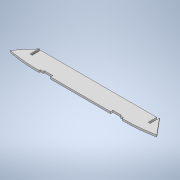
# Autodesk Inventor part: transom
Saved by Autodesk Inventor 2020.3 (Build 243373010, 373A)
## iProperties
Created: 2020-05-22
Part Number: transom
Material: Generic
Document SubType Name: Modeling
Designer: kardo
Density: 1 g/cm^3
Appearance: Default
Mass: 5.00225 g
Surface Area: 57.3573 cm^2
Volume: 5.00225 cm^3
Author: kardo
Autodesk Inventor part; units mm, degrees
ref_plane "YZ Plane" through (0, 0, 0) normal (1, 0, 0) x (0, 1, 0)
ref_plane "XZ Plane" through (0, 0, 0) normal (0, 1, 0) x (-1, 0, 0)
ref_plane "XY Plane" through (0, 0, 0) normal (0, 0, 1) x (1, 0, 0)
derived "base_sketch.ipt"
sketch "transom" plane through (0, -306, 31.875) normal (0, 1, 0) x (-1, 0, 0)
  line L0 (19.176, 14.943) -> (62.322, 14.943)
  line L1 (62.322, 14.943) -> (62.322, -18.346)
  line L2 (28.764, -18.346) -> (62.322, -18.346)
  line L3 (0, -18.5331) -> (-13.7575, -2.1376)
  line L4 (0, -18.5331) -> (0, -17.85)
  line L5 (0, -17.85) -> (62.322, -17.85)
  line L6 (62.322, 0.918) -> (19.176, 0.918)
  line L7 (19.176, 14.943) -> (19.176, 0.918) construction
  line L8 (-2.8595, -0.3503) -> (-2.8595, 13.6747) construction
  line L9 (-13.7575, 11.8874) -> (-13.7575, -2.1376) construction
  line L10 (8.1347, 14.7187) -> (8.1347, 0.6937) construction
  spline S0 degree 4 poles (-57.528, -4.335) (-46.0483, 2.3301) (-30.6129, 8.6531) (-11.2214, 13.1664) (8.3201, 14.943) (15.5662, 14.943) (19.176, 14.943) knots 0 0 0 0 0 0.630279 0.815816 1 1 1 1 1
  spline S1 degree 3 poles (19.176, 0.918) (8.1274, 1.1291) (-2.9238, -0.0043) (-13.7575, -2.1376) knots 0 0 0 0 1 1 1 1
  line L11 (0, 0) -> (0, -20.4)
  line L12 (0, 0) -> (0, 14.025) construction
  line L13 (-13.7575, 11.8874) -> (-2.8595, 13.6747) construction
  line L14 (-2.8595, 13.6747) -> (8.1347, 14.7187) construction
  line L15 (8.1347, 14.7187) -> (19.176, 14.943) construction
  point P0 (0, -31.875)
  point P1 (-38.352, -9.18)
  point P2 (-19.176, 10.7202)
  point P3 (-38.352, 4.845)
ref_plane "transom_plane" through (0, -306, 31.875) normal (0, 1, 0) x (-1, 0, 0)
sketch "Sketch2" plane through (0, -306, 31.875) normal (0, 1, 0) x (-1, 0, 0)
  line L0 (0, -18.5331) -> (-13.7575, -2.1376) projected
  line L1 (0, -17.85) -> (62.322, -17.85) projected
  line L2 (0, -20.4) -> (0, -17.85) projected
  spline S0 degree 3 poles (19.176, 0.918) (8.1274, 1.1291) (-2.9238, -0.0043) (-13.7575, -2.1376) knots 0 0 0 0 1 1 1 1 projected
  line L3 (62.322, 0.918) -> (19.176, 0.918) projected
  line L4 (62.322, 14.943) -> (62.322, -18.346) projected
  line L5 (0, -17.85) -> (0, -8.9267)
  line L6 (0, -8.9267) -> (2, -8.9267)
  line L7 (2, -8.9267) -> (2, -17.85)
  line L8 (0, -8.9267) -> (0, -0.0034) construction
  line L9 (19.176, 0.918) -> (19.176, -0.282)
  line L10 (19.176, -0.282) -> (22.176, -0.282)
  line L11 (22.176, -0.282) -> (25.176, -0.282) construction
  line L12 (25.176, -0.282) -> (25.176, 0.918) construction
  line L13 (22.176, -0.282) -> (22.176, -1.482)
  line L14 (22.176, -1.482) -> (31.176, -1.482)
  line L15 (31.176, -1.482) -> (31.176, 0.918)
  point P0 (0, -31.875)
  point P1 (-38.352, -9.18)
  dimension "d1" = 2
  dimension "d4" = 1.2
  dimension "d5" = 1.2
  dimension "d6" = 6
  dimension "d7" = 6
  constraints: 22 end point, 5 parallel, 4 collinear, 4 perpendicular, 3 point on line, 2 other
  measures "d1" distance of L5.end L6.end
  measures "d4" distance of L3.end L9.end
  measures "d5" distance of L10.end L13.end
  measures "d6" distance between parallel lines of L9 L12
  measures "d7" distance between parallel lines of L15 L12
extrude "Extrusion1" add sketch "Sketch2" along normal blind 2 contours L0 S0 L9 L10 L13 L14 L15 L3 L4 L1 L7 L6 L5 L2
mirror "Mirror1" about plane through (-62.322, -306, 14.025) normal (-1, 0, 0) of "Extrusion1"
equation "\"d1\" = stringer_thickness"
equation "\"d4\" = decking_thickness"
equation "\"d5\" = decking_thickness"
equation "\"d6\" = cowl_strip_width"
equation "\"d7\" = cowl_insulation_width"
equation "\"d2\" = bulkhead_thickness"
equation "\"stringer_thickness\" = 2"
equation "\"decking_thickness\" = 1.2"
equation "\"cowl_strip_width\" = 6"
equation "\"cowl_insulation_width\" = 6"
equation "\"bulkhead_thickness\" = 2"
body "Solid1"
